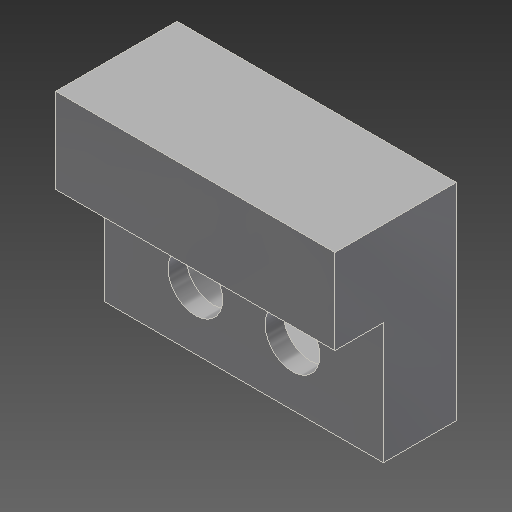
# Autodesk Inventor part: 05
Saved by Autodesk Inventor 2021.1 (Build 251245010, 245A)
## iProperties
Created: 2008-11-14
Part Number: 05
Document SubType Name: Modeling
Density: 8.08 g/cm^3
Material: SUS303
Mass: 31.1888 g
Surface Area: 18.32 cm^2
Volume: 3.86 cm^3
Appearance: 鋼
個数: 1
尺度: 2:1
Title: ブロック
Autodesk Inventor part; units mm, degrees
ref_plane "YZ Plane" through (0, 0, 0) normal (1, 0, 0) x (0, 1, 0)
ref_plane "XZ Plane" through (0, 0, 0) normal (0, 1, 0) x (-1, 0, 0)
ref_plane "XY Plane" through (0, 0, 0) normal (0, 0, 1) x (1, 0, 0)
sketch "スケッチ1" plane through (0, 0, 0) normal (0, 0, 1) x (1, 0, 0)
  line L0 (-11.5, 17) -> (11.5, 17)
  line L1 (11.5, 17) -> (11.5, 0)
  line L2 (11.5, 0) -> (-11.5, 0)
  line L3 (-11.5, 0) -> (-11.5, 17)
  point P0 (0, 0)
  point P1 (0, 0)
  dimension "d0" = 23
  dimension "d1" = 17
  constraints: 8 end point, 2 parallel, 1 coincident, 1 horizontal, 1 midpoint, 1 perpendicular
  measures "d0" distance of L1.end L2.end
  measures "d1" distance of L0.end L1.end
extrude "押し出し1" add sketch "スケッチ1" along normal blind 6
sketch "スケッチ5" plane through (0, 0, 0) normal (0, 0, -1) x (-1, 0, 0)
  line L0 (-11.5, 0) -> (11.5, 0) projected
  point P0 (0, 0)
  point P1 (-4, 5)
  point P2 (4, 5)
  dimension "d13" = 4
  dimension "d14" = 4
  dimension "d15" = 5
  constraints: 1 horizontal alignment
  measures "d13" horizontal distance of point (-4, 5) point (0, 0)
  measures "d14" horizontal distance of point (4, 5) point (0, 0)
  measures "d15" distance from line of point (-4, 5) L0
hole "穴1" at (4, 5, 0) at (-4, 5, 0) direction (0, 0, 1) diameter 4.5 end through all counterbore diameter 8 counterbore depth 4.5
sketch "スケッチ6" plane through (0, 0, 0) normal (0, 0, -1) x (-1, 0, 0)
  circle A0 centre (4, 5) radius 4 projected
  circle A1 centre (-4, 5) radius 4 projected
  line L0 (-4, 9) -> (4, 9)
  line L1 (-3.6249, 1.0176) -> (3.9907, 1)
  point P0 (0, 5)
  point P1 (0, 0)
  constraints: 4 end point, 4 point on circle, 3 tangent
extrude "押し出し5" cut sketch "スケッチ6" against normal up to surface (4.5 mm away) contours A0 A1 L0 | L1 A1 A0
sketch "スケッチ9" plane through (0, 0, 6) normal (0, 0, 1) x (1, 0, 0)
  line L0 (11.5, 17) -> (11.5, 0) projected
  line L1 (-11.5, 17) -> (11.5, 17) projected
  line L2 (-11.5, 0) -> (-11.5, 17) projected
  line L3 (11.5, 0) -> (-11.5, 0) projected
  line L4 (-11.5, 10) -> (11.5, 10)
  point P0 (0, 0)
  dimension "d32" = 10
  constraints: 2 end point, 2 point on line, 1 horizontal
  measures "d32" distance between parallel lines of L4 L3
extrude "押し出し8" add sketch "スケッチ9" along normal blind 4 contours L0 L4 L2 L1
equation "\"d14\" = d13"
